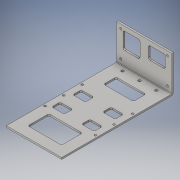
# Autodesk Inventor part: TempatBatteryRevisi2
Saved by Autodesk Inventor 2016 (Build 200138000, 138)
## iProperties
Created: 2017-04-24
Part Number: TempatBatteryRevisi2
Material: Generic
Document SubType Name: Modeling
Designer: Ghana
Density: 1 g/cm^3
Appearance: Default
Author: Ghana
Autodesk Inventor part; units mm, degrees
ref_plane "YZ Plane" through (0, 0, 0) normal (1, 0, 0) x (0, 1, 0)
ref_plane "XZ Plane" through (0, 0, 0) normal (0, 1, 0) x (-1, 0, 0)
ref_plane "XY Plane" through (0, 0, 0) normal (0, 0, 1) x (1, 0, 0)
sketch "Sketch1" plane through (0, 0, 0) normal (0, 1, 0) x (-1, 0, 0)
  line L0 (0, 0) -> (65.4, 0)
  line L1 (65.4, 0) -> (65.4, -130)
  line L2 (65.4, -130) -> (0, -130)
  line L3 (0, -130) -> (0, 0)
  line L4 (65.4, -130) -> (0, -130)
  line L5 (0, -130) -> (0, -132)
  line L6 (0, -132) -> (65.4, -132)
  line L7 (65.4, -132) -> (65.4, -130)
  line L8 (65.4, -132) -> (0, -132)
  line L9 (0, -132) -> (0, -172)
  line L10 (0, -172) -> (65.4, -172)
  line L11 (65.4, -172) -> (65.4, -132)
  circle A0 centre (62.6, -65) radius 1.3
  circle A1 centre (62.6, -43) radius 1.3
  circle A2 centre (62.6, -87) radius 1.3
  line L12 (48.4, -115) -> (17, -115)
  line L13 (15, -113) -> (15, -102)
  line L14 (17, -100) -> (48.4, -100)
  line L15 (50.4, -102) -> (50.4, -113)
  line L16 (44.9, -71) -> (55.9, -71)
  line L17 (57.9, -73) -> (57.9, -79)
  line L18 (55.9, -81) -> (44.9, -81)
  line L19 (42.9, -79) -> (42.9, -73)
  line L20 (42.9, -71) -> (57.9, -81) construction
  line L21 (57.9, -71) -> (42.9, -81) construction
  line L22 (44.9, -46) -> (55.9, -46)
  line L23 (57.9, -48) -> (57.9, -54)
  line L24 (55.9, -56) -> (44.9, -56)
  line L25 (42.9, -54) -> (42.9, -48)
  line L26 (42.9, -46) -> (57.9, -56) construction
  line L27 (57.9, -46) -> (42.9, -56) construction
  line L28 (14.7, -37.5) -> (50.7, -37.5)
  line L29 (52.7, -35.5) -> (52.7, -14.5)
  line L30 (50.7, -12.5) -> (14.7, -12.5)
  line L31 (12.7, -14.5) -> (12.7, -35.5)
  line L32 (12.7, -37.5) -> (52.7, -12.5) construction
  line L33 (52.7, -37.5) -> (12.7, -12.5) construction
  arc A3 (55.9, -81) -> (57.9, -79) centre (55.9, -79) ccw
  arc A4 (42.9, -79) -> (44.9, -81) centre (44.9, -79) ccw
  arc A5 (44.9, -71) -> (42.9, -73) centre (44.9, -73) ccw
  arc A6 (57.9, -73) -> (55.9, -71) centre (55.9, -73) ccw
  arc A7 (55.9, -56) -> (57.9, -54) centre (55.9, -54) ccw
  arc A8 (42.9, -54) -> (44.9, -56) centre (44.9, -54) ccw
  arc A9 (44.9, -46) -> (42.9, -48) centre (44.9, -48) ccw
  arc A10 (57.9, -48) -> (55.9, -46) centre (55.9, -48) ccw
  circle A11 centre (2.8, -65) radius 1.3
  circle A12 centre (2.8, -43) radius 1.3
  circle A13 centre (2.8, -87) radius 1.3
  line L34 (20.5, -71) -> (9.5, -71)
  line L35 (7.5, -73) -> (7.5, -79)
  line L36 (9.5, -81) -> (20.5, -81)
  line L37 (22.5, -79) -> (22.5, -73)
  line L38 (22.5, -71) -> (7.5, -81) construction
  line L39 (7.5, -71) -> (22.5, -81) construction
  line L40 (20.5, -46) -> (9.5, -46)
  line L41 (7.5, -48) -> (7.5, -54)
  line L42 (9.5, -56) -> (20.5, -56)
  line L43 (22.5, -54) -> (22.5, -48)
  line L44 (22.5, -46) -> (7.5, -56) construction
  line L45 (7.5, -46) -> (22.5, -56) construction
  arc A14 (7.5, -79) -> (9.5, -81) centre (9.5, -79) ccw
  arc A15 (20.5, -81) -> (22.5, -79) centre (20.5, -79) ccw
  arc A16 (22.5, -73) -> (20.5, -71) centre (20.5, -73) ccw
  arc A17 (9.5, -71) -> (7.5, -73) centre (9.5, -73) ccw
  arc A18 (7.5, -54) -> (9.5, -56) centre (9.5, -54) ccw
  arc A19 (20.5, -56) -> (22.5, -54) centre (20.5, -54) ccw
  arc A20 (22.5, -48) -> (20.5, -46) centre (20.5, -48) ccw
  arc A21 (9.5, -46) -> (7.5, -48) centre (9.5, -48) ccw
  arc A22 (50.4, -102) -> (48.4, -100) centre (48.4, -102) ccw
  arc A23 (48.4, -115) -> (50.4, -113) centre (48.4, -113) ccw
  arc A24 (15, -113) -> (17, -115) centre (17, -113) ccw
  arc A25 (17, -100) -> (15, -102) centre (17, -102) ccw
  arc A26 (52.7, -14.5) -> (50.7, -12.5) centre (50.7, -14.5) ccw
  arc A27 (50.7, -37.5) -> (52.7, -35.5) centre (50.7, -35.5) ccw
  arc A28 (12.7, -35.5) -> (14.7, -37.5) centre (14.7, -35.5) ccw
  arc A29 (14.7, -12.5) -> (12.7, -14.5) centre (14.7, -14.5) ccw
  circle A30 centre (12.7, -125) radius 1.6
  circle A31 centre (32.7, -125) radius 1.6
  circle A32 centre (52.7, -125) radius 1.6
  line L46 (55.7, -167) -> (39.7, -167)
  line L47 (37.7, -165) -> (37.7, -149)
  line L48 (39.7, -147) -> (55.7, -147)
  line L49 (57.7, -149) -> (57.7, -165)
  line L50 (57.7, -167) -> (37.7, -147) construction
  line L51 (37.7, -167) -> (57.7, -147) construction
  arc A33 (55.7, -167) -> (57.7, -165) centre (55.7, -165) ccw
  arc A34 (37.7, -165) -> (39.7, -167) centre (39.7, -165) ccw
  arc A35 (39.7, -147) -> (37.7, -149) centre (39.7, -149) ccw
  arc A36 (57.7, -149) -> (55.7, -147) centre (55.7, -149) ccw
  line L52 (9.7, -167) -> (25.7, -167)
  line L53 (27.7, -165) -> (27.7, -154)
  line L54 (25.7, -152) -> (9.7, -152)
  line L55 (7.7, -154) -> (7.7, -165)
  line L56 (7.7, -167) -> (27.7, -152) construction
  line L57 (27.7, -167) -> (7.7, -152) construction
  arc A37 (7.7, -165) -> (9.7, -167) centre (9.7, -165) ccw
  arc A38 (25.7, -167) -> (27.7, -165) centre (25.7, -165) ccw
  arc A39 (27.7, -154) -> (25.7, -152) centre (25.7, -154) ccw
  arc A40 (9.7, -152) -> (7.7, -154) centre (9.7, -154) ccw
  line L58 (65.4, -172) -> (0, -172)
  point P0 (15, -100)
  point P1 (15, -115)
  dimension "d205" = 130
  dimension "d206" = 2
  dimension "d207" = 40
  dimension "d211" = 2.6
  dimension "d212" = 22
  dimension "d213" = 2.8
  dimension "d214" = 65
  dimension "d215" = 22
  dimension "d220" = 15
  dimension "d222" = 15
  dimension "d223" = 10
  dimension "d225" = 15
  dimension "d226" = 10
  dimension "d228" = 40
  dimension "d229" = 25
  dimension "d230" = 2
  dimension "d231" = 2
  dimension "d238" = 3.2
  dimension "d240" = 20
  dimension "d241" = 20
  dimension "d242" = 2
  dimension "d263" = 5
  dimension "d264" = 5
  dimension "d266" = 20
  constraints: 118 end point, 64 point on circle, 60 point on line, 41 centre point, 40 tangent, 19 equal radius, 16 parallel, 9 horizontal, 8 perpendicular, 2 vertical alignment
  measures "d205" distance of L0.end L1.end
  measures "d206" distance of L5.end L4.end
  measures "d207" distance of L9.end L8.end
  measures "d211" diameter of A0
  measures "d212" distance of A0.centre A2.centre
  measures "d213" distance from line of L1 A0.centre
  measures "d214" distance from line of L0 A0.centre
  measures "d215" distance of A0.centre A1.centre
  measures "d220" distance of point (15, -115) point (15, -100)
  measures "d222" distance of L20.end L21.end
  measures "d223" distance of L21.start L20.end
  measures "d225" distance of L26.end L27.end
  measures "d226" distance of L27.start L26.end
  measures "d228" distance of L33.end L32.end
  measures "d229" distance of L32.end L33.start
  measures "d230" radius of A3
  measures "d231" radius of A22
  measures "d238" diameter of A30
  measures "d240" distance of L50.end L51.end
  measures "d241" distance of L51.start L50.end
  measures "d242" radius of A33
  measures "d263" distance between parallel lines of L46 L58
  measures "d264" distance between parallel lines of L52 L58
  measures "d266" distance between parallel lines of L55 L53
extrude "Extrusion9" add sketch "Sketch1" along normal blind 2
sketch "Sketch19" plane through (0, 2, 0) normal (0, 1, 0) x (1, 0, 0)
  arc A0 (-50.7, 37.5) -> (-52.7, 35.5) centre (-50.7, 35.5) ccw projected
  line L0 (-50.7, 37.5) -> (-14.7, 37.5) projected
  arc A1 (-12.7, 35.5) -> (-14.7, 37.5) centre (-14.7, 35.5) ccw projected
  line L1 (-12.7, 35.5) -> (-12.7, 14.5) projected
  arc A2 (-14.7, 12.5) -> (-12.7, 14.5) centre (-14.7, 14.5) ccw projected
  line L2 (-14.7, 12.5) -> (-50.7, 12.5) projected
  arc A3 (-52.7, 14.5) -> (-50.7, 12.5) centre (-50.7, 14.5) ccw projected
  line L3 (-52.7, 14.5) -> (-52.7, 35.5) projected
  arc A4 (-48.4, 115) -> (-50.4, 113) centre (-48.4, 113) ccw projected
  line L4 (-48.4, 115) -> (-17, 115) projected
  arc A5 (-15, 113) -> (-17, 115) centre (-17, 113) ccw projected
  line L5 (-15, 113) -> (-15, 102) projected
  arc A6 (-17, 100) -> (-15, 102) centre (-17, 102) ccw projected
  line L6 (-17, 100) -> (-48.4, 100) projected
  arc A7 (-50.4, 102) -> (-48.4, 100) centre (-48.4, 102) ccw projected
  line L7 (-50.4, 102) -> (-50.4, 113) projected
  arc A8 (-22.5, 48) -> (-20.5, 46) centre (-20.5, 48) ccw projected
  line L8 (-22.5, 48) -> (-22.5, 54) projected
  arc A9 (-20.5, 56) -> (-22.5, 54) centre (-20.5, 54) ccw projected
  line L9 (-20.5, 56) -> (-9.5, 56) projected
  arc A10 (-7.5, 54) -> (-9.5, 56) centre (-9.5, 54) ccw projected
  line L10 (-7.5, 54) -> (-7.5, 48) projected
  arc A11 (-9.5, 46) -> (-7.5, 48) centre (-9.5, 48) ccw projected
  line L11 (-9.5, 46) -> (-20.5, 46) projected
  arc A12 (-7.5, 79) -> (-9.5, 81) centre (-9.5, 79) ccw projected
  line L12 (-7.5, 79) -> (-7.5, 73) projected
  arc A13 (-9.5, 71) -> (-7.5, 73) centre (-9.5, 73) ccw projected
  line L13 (-9.5, 71) -> (-20.5, 71) projected
  arc A14 (-22.5, 73) -> (-20.5, 71) centre (-20.5, 73) ccw projected
  line L14 (-22.5, 73) -> (-22.5, 79) projected
  arc A15 (-20.5, 81) -> (-22.5, 79) centre (-20.5, 79) ccw projected
  line L15 (-20.5, 81) -> (-9.5, 81) projected
  arc A16 (-42.9, 54) -> (-44.9, 56) centre (-44.9, 54) ccw projected
  line L16 (-42.9, 54) -> (-42.9, 48) projected
  arc A17 (-44.9, 46) -> (-42.9, 48) centre (-44.9, 48) ccw projected
  line L17 (-44.9, 46) -> (-55.9, 46) projected
  arc A18 (-57.9, 48) -> (-55.9, 46) centre (-55.9, 48) ccw projected
  line L18 (-57.9, 48) -> (-57.9, 54) projected
  arc A19 (-55.9, 56) -> (-57.9, 54) centre (-55.9, 54) ccw projected
  line L19 (-55.9, 56) -> (-44.9, 56) projected
  arc A20 (-42.9, 79) -> (-44.9, 81) centre (-44.9, 79) ccw projected
  line L20 (-42.9, 79) -> (-42.9, 73) projected
  arc A21 (-44.9, 71) -> (-42.9, 73) centre (-44.9, 73) ccw projected
  line L21 (-44.9, 71) -> (-55.9, 71) projected
  arc A22 (-57.9, 73) -> (-55.9, 71) centre (-55.9, 73) ccw projected
  line L22 (-57.9, 73) -> (-57.9, 79) projected
  arc A23 (-55.9, 81) -> (-57.9, 79) centre (-55.9, 79) ccw projected
  line L23 (-55.9, 81) -> (-44.9, 81) projected
  circle A24 centre (-52.7, 125) radius 1.6 projected
  circle A25 centre (-32.7, 125) radius 1.6 projected
  circle A26 centre (-12.7, 125) radius 1.6 projected
  circle A27 centre (-2.8, 43) radius 1.3 projected
  circle A28 centre (-2.8, 87) radius 1.3 projected
  circle A29 centre (-2.8, 65) radius 1.3 projected
  circle A30 centre (-62.6, 87) radius 1.3 projected
  circle A31 centre (-62.6, 43) radius 1.3 projected
  circle A32 centre (-62.6, 65) radius 1.3 projected
  arc A33 (-25.7, 167) -> (-27.7, 165) centre (-25.7, 165) ccw projected
  line L24 (-25.7, 167) -> (-9.7, 167) projected
  arc A34 (-7.7, 165) -> (-9.7, 167) centre (-9.7, 165) ccw projected
  line L25 (-7.7, 165) -> (-7.7, 154) projected
  arc A35 (-9.7, 152) -> (-7.7, 154) centre (-9.7, 154) ccw projected
  line L26 (-9.7, 152) -> (-25.7, 152) projected
  arc A36 (-27.7, 154) -> (-25.7, 152) centre (-25.7, 154) ccw projected
  line L27 (-27.7, 154) -> (-27.7, 165) projected
  arc A37 (-37.7, 165) -> (-39.7, 167) centre (-39.7, 165) ccw projected
  line L28 (-37.7, 165) -> (-37.7, 149) projected
  arc A38 (-39.7, 147) -> (-37.7, 149) centre (-39.7, 149) ccw projected
  line L29 (-39.7, 147) -> (-55.7, 147) projected
  arc A39 (-57.7, 149) -> (-55.7, 147) centre (-55.7, 149) ccw projected
  line L30 (-57.7, 149) -> (-57.7, 165) projected
  arc A40 (-55.7, 167) -> (-57.7, 165) centre (-55.7, 165) ccw projected
  line L31 (-55.7, 167) -> (-39.7, 167) projected
  line L32 (0, 0) -> (0, 172) projected
  line L33 (0, 172) -> (-65.4, 172) projected
  line L34 (-65.4, 172) -> (-65.4, 0) projected
  line L35 (-65.4, 0) -> (0, 0) projected
  line L36 (0, 0) -> (0, 172) projected
  line L37 (-65.4, 0) -> (0, 0)
  line L38 (0, 0) -> (0, 130)
  line L39 (0, 130) -> (-65.4, 130)
  line L40 (-65.4, 130) -> (-65.4, 0)
  dimension "d260" = 130
  constraints: 8 end point, 2 parallel, 1 horizontal, 1 perpendicular, 1 point on line
  measures "d260" distance of L38.end L37.end
bend part "Bend Part16" radius 0.6366 angle 90 line through (0, 2, -130) along (-1, 0, 0) centre toward (0, 1, 0) moving side (0, 0, -1) both sides no
sketch "Sketch21" plane through (0, 2.6366, -132.6366) normal (0, 0, -1) x (-1, 0, 0)
  line L0 (0, 0) -> (65.4, 0) projected
  line L1 (65.4, 41) -> (65.4, 0) projected
  line L2 (0, 41) -> (65.4, 41) projected
  line L3 (0, 0) -> (0, 41) projected
  arc A0 (39.7, 36) -> (37.7, 34) centre (39.7, 34) ccw projected
  line L4 (39.7, 36) -> (55.7, 36) projected
  arc A1 (57.7, 34) -> (55.7, 36) centre (55.7, 34) ccw projected
  line L5 (57.7, 34) -> (57.7, 18) projected
  arc A2 (55.7, 16) -> (57.7, 18) centre (55.7, 18) ccw projected
  line L6 (55.7, 16) -> (39.7, 16) projected
  arc A3 (37.7, 18) -> (39.7, 16) centre (39.7, 18) ccw projected
  line L7 (37.7, 18) -> (37.7, 34) projected
  arc A4 (27.7, 34) -> (25.7, 36) centre (25.7, 34) ccw projected
  line L8 (27.7, 34) -> (27.7, 23) projected
  arc A5 (25.7, 21) -> (27.7, 23) centre (25.7, 23) ccw projected
  line L9 (25.7, 21) -> (9.7, 21) projected
  arc A6 (7.7, 23) -> (9.7, 21) centre (9.7, 23) ccw projected
  line L10 (7.7, 23) -> (7.7, 34) projected
  arc A7 (9.7, 36) -> (7.7, 34) centre (9.7, 34) ccw projected
  line L11 (9.7, 36) -> (25.7, 36) projected
  line L12 (0, 0) -> (0, 41) projected
  circle A8 centre (5, 5) radius 1.3
  circle A9 centre (60.4, 5) radius 1.3
  circle A10 centre (5, 36) radius 1.3
  circle A11 centre (60.4, 36) radius 1.3
  point P0 (0, -2.6366)
  dimension "d272" = 2.6
  dimension "d273" = 2.6
  constraints: 4 centre point, 4 coincident
  measures "d272" diameter of A8
  measures "d273" diameter of A9
hole "Hole2" at (-5, 38.6366, -132.6366) at (-5, 7.6366, -132.6366) at (-60.4, 7.6366, -132.6366) at (-60.4, 38.6366, -132.6366) direction (0, 0, 1) diameter 2.6 end through all
body "Solid9"
